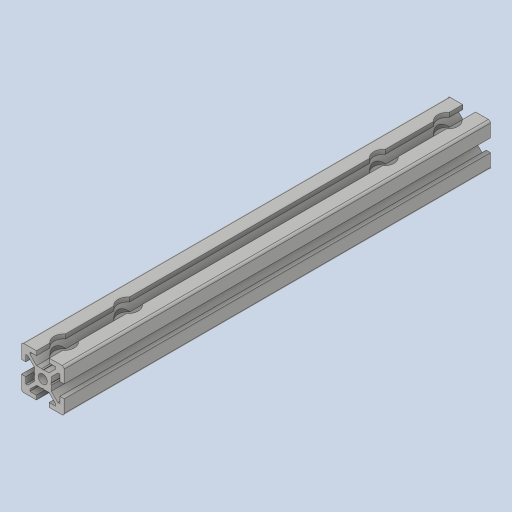
# Autodesk Inventor part: HFS5-2020-200-Z5-XA10-XB40-XC160-XD190
Saved by Autodesk Inventor 2023 (Build 270158000, 158)
## iProperties
Created: 2024-11-09
Part Number: HFS5-2020-200-Z5-XA10-XB40-XC160-XD190
Material: Generic
Catalog Web Link: www.cadenas.de
Description: NFS5-2020, NFSB5-2020, HFS5-2020, HFSB5-2020, CAF5-2020, HFSY5-2020, NFSF5-2020, HFSF5-2020, HFSFB5-2020, NFST5-2020, HFST5-2020, HFSTB5-2020, HFSH5-2020, HFSC5-2020-HFS5 Series Aluminum Extrusions 20 Square -1 Slot-
Vendor: MISUMI
Document SubType Name: Modeling
Designer: psAdmin
Manufacturer: MISUMI
Mass: 35.7548 g
Surface Area: 350.338 cm^2
Volume: 35.7548 cm^3
Density: 1 g/cm^3
Appearance: PSOLRGB-175-175-175
Category: PARTsolutions
Company: MISUMI
PSOL_IDENT_0: {$CADENAS_DATA/23d-libs/misumi/metric/38_al_extrusions_blackets/5/hfs5_2020.prj},727 {VTYP=3D},{NB=H
PSOL_IDENT_1: FS5-2020-200-Z5-XA10-XB40-XC160-XD190},{LINA=HFS5-2020-200-Z5-XA10-XB40-XC160-XD190},{NN=NFS5-2020,
PSOL_IDENT_2: NFSB5-2020, HFS5-2020, HFSB5-2020, CAF5-2020, HFSY5-2020, NFSF5-2020, HFSF5-2020, HFSFB5-2020, NFST5
PSOL_IDENT_3: -2020, HFST5-2020, HFSTB5-2020, HFSH5-2020, HFSC5-2020},{DATE=08.05.2023 08:39:06},{GEOMDATE=27.07.2
PSOL_IDENT_4: 021 03:20:00},{VERSION=},{LINEID=150},{WBVAR=L,ALT1,ALT2,ALT4,ALT5,CP5,DL5,DR5,ALT6,ALT9,ALT10,ALT11
PSOL_IDENT_5: ,HP6,NHL6,DL6,NHR6,DR6,ALT7,ALT8,NH9,AH,BH,CH,DH,EH,NH10,AV,BV,CV,DV,EV,NH11,AP,BP,CP,DP,EP,ALT12,AL
PSOL_IDENT_6: T13,Z,NH12,XA,XB,XC,XD,XE,NH13,YA,YB,YC,YD,YE,ALT16,HP16,DL16,DR16,ALT17,HQ17,JLP,ALT20},{WBNUMERIC=
PSOL_IDENT_7: L,NH9,AH,BH,CH,DH,EH,NH10,AV,BV,CV,DV,EV,NH11,AP,BP,CP,DP,EP,NH12,XA,XB,XC,XD,XE,NH13,YA,YB,YC,YD,YE
PSOL_IDENT_8: ,HQ17,JLP}  {NB=HFS5-2020-200-Z5-XA10-XB40-XC160-XD190},{LINA=HFS5-2020-200-Z5-XA10-XB40-XC160-XD190
PSOL_IDENT_9: },{KT=DUMMY},{PN=HFS5-2020-200-Z5-XA10-XB40-XC160-XD190},{TPS=HFS5-2020},{MAT=A6N01SS-T5 Aluminum Al
PSOL_IDENT_10: loy or 6005A-T5 Aluminum Alloy},{ST=Clear Anodize},{FRMW=20},{FRMH=20},{FRD=4.2},{L=200},{MASS=0.5},
PSOL_IDENT_11: {SA=183},{LX=0.742x10^4},{LY=0.742x10^4},{ALT1=},{M1=0},{DPL1=0},{DPR1=0},{ALT1PN=},{ALT2=},{ALT2ALG=
PSOL_IDENT_12: '','w/o End Tapping (Heli-Coil Insert)','LHP','with LHP (Tapping on the Left (Heli-Coil Insert))','
PSOL_IDENT_13: RHP','with RHP (Tapping on the Right (Heli-Coil Insert))','HPW','with HPW (Tapping on Both Ends (Hel
PSOL_IDENT_14: i-Coil Insert))' },{M2=0},{DP2=0},{ALT2PN=},{ALT4=},{ALT4ALG= '', 'w/o SC (High Precision Cut)', 'SC'
PSOL_IDENT_15: , 'with SC (High Precision Cut)' },{ALT4PN=},{ALT5=},{ALT5ALG= '','w/o 45 Degree Cut','1','with 45 D
PSOL_IDENT_16: egree Cut' },{CP5=},{CP5ALG= '','N/A' },{DL5=},{DL5ALG= '','N/A' },{DR5=},{DR5ALG= '','N/A' },{FRMLA
PSOL_IDENT_17: LT5=0},{FRMRALT5=0},{ALT5PN=},{ALT6=},{ALT6ALG= '','w/o Fastening Location Wrench Access Hole Altera
PSOL_IDENT_18: tions','1','with Fastening Location Wrench Access Hole Alterations' },{ALT9=},{ALT9ALG= '','w/o Loca
PSOL_IDENT_19: tion Specified Wrench Access Hole Alteratons (Horizontal)','1','with Location Specified Wrench Acces
PSOL_IDENT_20: s Hole Alteratons (Horizontal)' },{ALT10=},{ALT10ALG= '','w/o Location Specified Wrench Access Hole
PSOL_IDENT_21: Alteratons (Vertical)','1','with Location Specified Wrench Access Hole Alteratons (Vertical)' },{ALT
PSOL_IDENT_22: 11=},{ALT11ALG= '','w/o Location Specified Wrench Access Hole Alteratons (Crisscross)','1','with Loc
PSOL_IDENT_23: ation Specified Wrench Access Hole Alteratons (Crisscross)' },{HP6=},{HP6ALG= '','N/A' },{NHL6=},{NH
PSOL_IDENT_24: L6ALG= '','N/A' },{DL6=},{DL6ALG= '','N/A' },{NHR6=},{NHR6ALG= '','N/A' },{DR6=},{DR6ALG= '','N/A' }
PSOL_IDENT_25: ,{HL6=0.000},{HL6D=0},{HR6=0.000},{HR6D=0},{J6=0},{J6D=0},{K6=0},{K6D=0},{DD6=0.00},{DD6ALG=0},{ALT7=
PSOL_IDENT_26: },{ALT7ALG= '','N/A' },{ALT8=},{ALT8ALG= '','N/A' },{ALT678PN=},{NH9=0},{NH9MAX=5},{NH9ALG=[0]},{AH=
PSOL_IDENT_27: 0.0},{AHMIN=7},{AHMAX=195},{AHALG=[0]},{BH=0.0},{BHMIN=2},{BHMAX=197},{BHALG=[0]},{CH=0.0},{CHMIN=2}
PSOL_IDENT_28: ,{CHMAX=199},{CHALG=[0]},{DH=0.0},{DHMIN=2},{DHMAX=201},{DHALG=[0]},{EH=0.0},{EHMIN=2},{EHMAX=193},{
PSOL_IDENT_29: EHALG=[0]},{NH10=0},{NH10MAX=5},{NH10ALG=[0]},{AV=0.0},{AVMIN=7},{AVMAX=195},{AVALG=[0]},{BV=0.0},{B
PSOL_IDENT_30: VMIN=2},{BVMAX=197},{BVALG=[0]},{CV=0.0},{CVMIN=2},{CVMAX=199},{CVALG=[0]},{DV=0.0},{DVMIN=2},{DVMAX=
PSOL_IDENT_31: 201},{DVALG=[0]},{EV=0.0},{EVMIN=2},{EVMAX=193},{EVALG=[0]},{NH11=0},{NH11MAX=5},{NH11ALG=[0]},{AP=0
PSOL_IDENT_32: .0},{APMIN=7},{APMAX=195},{APALG=[0]},{BP=0.0},{BPMIN=2},{BPMAX=197},{BPALG=[0]},{CP=0.0},{CPMIN=2},
PSOL_IDENT_33: {CPMAX=199},{CPALG=[0]},{DP=0.0},{DPMIN=2},{DPMAX=201},{DPALG=[0]},{EP=0.0},{EPMIN=2},{EPMAX=193},{E
PSOL_IDENT_34: PALG=[0]},{ALT9PN=},{ALT10PN=},{ALT11PN=},{ALT91011PN=},{ALT12=1},{ALT12ALG= '','w/o Counterbore Hol
PSOL_IDENT_35: e in Specified Position (Vertical)','1','with Counterbore Hole in Specified Position (Vertical)' },{
PSOL_IDENT_36: ALT13=},{ALT13ALG= '','w/o Counterbore Hole in Specified Position (Horizontal)','1','with Counterbor
PSOL_IDENT_37: e Hole in Specified Position (Horizontal)' },{Z=5},{ZALG='5','5','6','6'},{DD12=5.5},{DD112=9.5},{NH
PSOL_IDENT_38: 12=4},{NH12MAX=5},{NH12ALG=[1:5/1]},{XA=10.0},{XAMIN=7},{XAMAX=158.5},{XAALG=[7:158.5/0.5]},{XB=40.0
PSOL_IDENT_39: },{XBMIN=21.5},{XBMAX=170},{XBALG=[21.5:170/0.5]},{XC=160.0},{XCMIN=51.5},{XCMAX=181.5},{XCALG=[51.5
PSOL_IDENT_40: :181.5/0.5]},{XD=190.0},{XDMIN=171.5},{XDMAX=193},{XDALG=[171.5:193/0.5]},{XE=0.0},{XEMIN=201.5},{XE
PSOL_IDENT_41: MAX=193},{XEALG=[0]},{NH13=0},{NH13MAX=5},{NH13ALG=[0]},{YA=0.0},{YAMIN=7},{YAMAX=204.5},{YAALG=[0]}
PSOL_IDENT_42: ,{YB=0.0},{YBMIN=11.5},{YBMAX=216},{YBALG=[0]},{YC=0.0},{YCMIN=11.5},{YCMAX=227.5},{YCALG=[0]},{YD=0
PSOL_IDENT_43: .0},{YDMIN=11.5},{YDMAX=239},{YDALG=[0]},{YE=0.0},{YEMIN=11.5},{YEMAX=193},{YEALG=[0]},{ALT12PN=-XA1
PSOL_IDENT_44: 0-XB40-XC160-XD190},{ALT13PN=},{ALT1213PN=-Z5-XA10-XB40-XC160-XD190},{ALT16=},{ALT16ALG= '','w/o M T
PSOL_IDENT_45: ype Hole Alteration','1','with M Type Hole Alteration' },{HP16=},{HP16ALG= '','N/A' },{DL16=},{DL16A
PSOL_IDENT_46: LG= '','N/A' },{DR16=},{DR16ALG= '','N/A' },{H116=0},{D16=0.0},{ALT16PN=},{ALT17=},{ALT17ALG= '','w/
PSOL_IDENT_47: o L Type Hole Alteration (Top)','1','with L Type Hole Alteration (Top)' },{HQ17=0},{HQ17ALG=0},{JLP=
PSOL_IDENT_48: 0},{JLPMIN=4.9},{JLPMAX=0},{JLPALG=[0]},{L17=0},{D17=0.0},{ALT17PN=},{ALT20=},{ALT20PN=},{ERRORALT01=
PSOL_IDENT_49: OK},{ERRORALT02=OK},{ERRORALT05=OK},{ERRORALT06091=OK},{ERRORALT06092=OK},{ERRORALT06093=OK},{ERRORA
PSOL_IDENT_50: LT06094=OK},{ERRORALT06101=OK},{ERRORALT06102=OK},{ERRORALT06103=OK},{ERRORALT06104=OK},{ERRORALT061
PSOL_IDENT_51: 11=OK},{ERRORALT06112=OK},{ERRORALT06113=OK},{ERRORALT06114=OK},{ERRORALT06121=OK},{ERRORALT06122=OK
PSOL_IDENT_52: },{ERRORALT06123=OK},{ERRORALT06124=OK},{ERRORALT06131=OK},{ERRORALT06132=OK},{ERRORALT06133=OK},{ER
PSOL_IDENT_53: RORALT06134=OK},{ERRORALT0616=OK},{ERRORALT06171=OK},{ERRORALT06172=OK},{ERRORALT06173=OK},{ERRORALT
PSOL_IDENT_54: 0911=OK},{ERRORALT0913=OK},{ERRORALT0916=OK},{ERRORALT0917=OK},{ERRORALT1011=OK},{ERRORALT1012=OK},{
PSOL_IDENT_55: ERRORALT1016=OK},{ERRORALT1017=OK},{ERRORALT1112=OK},{ERRORALT1113=OK},{ERRORALT1116=OK},{ERRORALT11
PSOL_IDENT_56: 17=OK},{ERRORALT1216=OK},{ERRORALT1217=OK},{ERRORALT1316=OK},{ERRORALT1317=OK},{ERRORALT1617=OK},{ER
PSOL_IDENT_57: RORPN=},{TFW=0}
NB: HFS5-2020-200-Z5-XA10-XB40-XC160-XD190
NN: NFS5-2020, NFSB5-2020, HFS5-2020, HFSB5-2020, CAF5-2020, HFSY5-2020, NFSF5-2020, HFSF5-2020, HFSFB5-2020, NFST5-2020, HFST5-2020, HFSTB5-2020, HFSH5-2020, HFSC5-2020
NT: HFS5 Series Aluminum Extrusions 20 Square -1 Slot-
NBSYN: $PN.
LINA: HFS5-2020-200-Z5-XA10-XB40-XC160-XD190
CATALOG: Misumi
PN: HFS5-2020-200-Z5-XA10-XB40-XC160-XD190
TPS: HFS5-2020
MAT: A6N01SS-T5 Aluminum Alloy or 6005A-T5 Aluminum Alloy
ST: Clear Anodize
L: 200
MASS: 0.5
SA: 183
LX: 0.742x10^4
LY: 0.742x10^4
ALT1: w/o End Tapping
M1: 0
DPL1: 0
DPR1: 0
ALT2: w/o End Tapping (Heli-Coil Insert)
M2: 0
DP2: 0
ALT4: w/o SC (High Precision Cut)
ALT5: w/o 45 Degree Cut
CP5: N/A
DL5: N/A
DR5: N/A
ALT6: w/o Fastening Location Wrench Access Hole Alterations
ALT9: w/o Location Specified Wrench Access Hole Alteratons (Horizontal)
ALT10: w/o Location Specified Wrench Access Hole Alteratons (Vertical)
ALT11: w/o Location Specified Wrench Access Hole Alteratons (Crisscross)
HP6: N/A
NHL6: N/A
DL6: N/A
NHR6: N/A
DR6: N/A
HL6D: 0
HR6D: 0
J6D: 0
K6D: 0
DD6: 0
ALT7: N/A
ALT8: N/A
NH9: 0
AH: 0
BH: 0
CH: 0
DH: 0
EH: 0
NH10: 0
AV: 0
BV: 0
CV: 0
DV: 0
EV: 0
NH11: 0
AP: 0
BP: 0
CP: 0
DP: 0
EP: 0
ALT12: with Counterbore Hole in Specified Position (Vertical)
ALT13: w/o Counterbore Hole in Specified Position (Horizontal)
Z: 5
DD12: 5.5
DD112: 9.5
NH12: 4
XA: 10
XB: 40
XC: 160
XD: 190
XE: 0
NH13: 0
YA: 0
YB: 0
YC: 0
YD: 0
YE: 0
ALT16: w/o M Type Hole Alteration
HP16: N/A
DL16: N/A
DR16: N/A
H116: 0
D16: 0
ALT17: w/o L Type Hole Alteration (Top)
HQ17: 0
JLP: 0
D17: 0
ALT20: w/o CW (End Face C Chamfering)
SUPPLIER: MISUMI
ARTICLENO: HFS5-2020-200-Z5-XA10-XB40-XC160-XD190
BOMINFO: HFS5-2020-200-Z5-XA10-XB40-XC160-XD190
CREATOR: CADENAS GmbH
Title: HFS5-2020-200-Z5-XA10-XB40-XC160-XD190
Author: Cadenas PARTsolutions
Comments: HFS5 Series Aluminum Extrusions 20 Square -1 Slot-
Autodesk Inventor part; units mm, degrees
sketch "Sketch_1" plane through (0, 0, 0) normal (0, 0, 1) x (1, 0, 0)
  line L0 (-10, -3) -> (-10, -9)
  arc A0 (-10, -9) -> (-9, -10) centre (-9, -9) ccw
  line L1 (-9, -10) -> (-3, -10)
  line L2 (-3, -10) -> (-3, -8)
  line L3 (-3, -8) -> (-6, -8)
  line L4 (-6, -8) -> (-6, -7.0607)
  line L5 (-6, -7.0607) -> (-2.9393, -4)
  line L6 (-2.9393, -4) -> (-0.5196, -4)
  line L7 (-0.5196, -4) -> (0, -3.7)
  line L8 (0, -3.7) -> (0.5196, -4)
  line L9 (0.5196, -4) -> (2.9393, -4)
  line L10 (2.9393, -4) -> (6, -7.0607)
  line L11 (6, -7.0607) -> (6, -8)
  line L12 (6, -8) -> (3, -8)
  line L13 (3, -8) -> (3, -10)
  line L14 (3, -10) -> (9, -10)
  arc A1 (9, -10) -> (10, -9) centre (9, -9) ccw
  line L15 (10, -9) -> (10, -3)
  line L16 (10, -3) -> (8, -3)
  line L17 (8, -3) -> (8, -6)
  line L18 (8, -6) -> (7.0607, -6)
  line L19 (7.0607, -6) -> (4, -2.9393)
  line L20 (4, -2.9393) -> (4, -0.5196)
  line L21 (4, -0.5196) -> (3.7, 0)
  line L22 (3.7, 0) -> (4, 0.5196)
  line L23 (4, 0.5196) -> (4, 2.9393)
  line L24 (4, 2.9393) -> (7.0607, 6)
  line L25 (7.0607, 6) -> (8, 6)
  line L26 (8, 6) -> (8, 3)
  line L27 (8, 3) -> (10, 3)
  line L28 (10, 3) -> (10, 9)
  arc A2 (10, 9) -> (9, 10) centre (9, 9) ccw
  line L29 (9, 10) -> (3, 10)
  line L30 (3, 10) -> (3, 8)
  line L31 (3, 8) -> (6, 8)
  line L32 (6, 8) -> (6, 7.0607)
  line L33 (6, 7.0607) -> (2.9393, 4)
  line L34 (2.9393, 4) -> (0.5196, 4)
  line L35 (0.5196, 4) -> (0, 3.7)
  line L36 (0, 3.7) -> (-0.5196, 4)
  line L37 (-0.5196, 4) -> (-2.9393, 4)
  line L38 (-2.9393, 4) -> (-6, 7.0607)
  line L39 (-6, 7.0607) -> (-6, 8)
  line L40 (-6, 8) -> (-3, 8)
  line L41 (-3, 8) -> (-3, 10)
  line L42 (-3, 10) -> (-9, 10)
  arc A3 (-9, 10) -> (-10, 9) centre (-9, 9) ccw
  line L43 (-10, 9) -> (-10, 3)
  line L44 (-10, 3) -> (-8, 3)
  line L45 (-8, 3) -> (-8, 6)
  line L46 (-8, 6) -> (-7.0607, 6)
  line L47 (-7.0607, 6) -> (-4, 2.9393)
  line L48 (-4, 2.9393) -> (-4, 0.5196)
  line L49 (-4, 0.5196) -> (-3.7, 0)
  line L50 (-3.7, 0) -> (-4, -0.5196)
  line L51 (-4, -0.5196) -> (-4, -2.9393)
  line L52 (-4, -2.9393) -> (-7.0607, -6)
  line L53 (-7.0607, -6) -> (-8, -6)
  line L54 (-8, -6) -> (-8, -3)
  line L55 (-8, -3) -> (-10, -3)
  constraints: 112 end point, 8 point on circle, 4 centre point
extrude "Extrusion1" add sketch "Sketch_1" against normal blind 200
sketch "Sketch2" plane through (0, 0, -200) normal (0, 0, -1) x (-1, 0, 0)
  point P0 (0, 0)
hole "Hole1" at (0, 0, -200) direction (0, 0, 1) diameter 4.2 depth 200
sketch "Sketch_30" plane through (0, 0, 0) normal (1, 0, 0) x (0, 0, -1)
  line L0 (10, -10) -> (10, 10)
  line L1 (10, 10) -> (14.75, 10)
  line L2 (14.75, 10) -> (14.75, 4)
  line L3 (14.75, 4) -> (12.75, 4)
  line L4 (12.75, 4) -> (12.75, -10)
  line L5 (12.75, -10) -> (10, -10)
  line L6 (10, -10) -> (10, 10)
  constraints: 14 end point
revolve "Revolution1" cut sketch "Sketch_30" angle 360 about axis through (0, -10, -10) along (0, -1, 0)
sketch "Sketch_31" plane through (0, 0, 0) normal (1, 0, 0) x (0, 0, -1)
  line L0 (40, -10) -> (40, 10)
  line L1 (40, 10) -> (44.75, 10)
  line L2 (44.75, 10) -> (44.75, 4)
  line L3 (44.75, 4) -> (42.75, 4)
  line L4 (42.75, 4) -> (42.75, -10)
  line L5 (42.75, -10) -> (40, -10)
  line L6 (40, -10) -> (40, 10)
  constraints: 14 end point
revolve "Revolution2" cut sketch "Sketch_31" angle 360 about axis through (0, -10, -40) along (0, -1, 0)
sketch "Sketch_47" plane through (0, 0, 0) normal (1, 0, 0) x (0, 0, -1)
  line L0 (160, -10) -> (160, 10)
  line L1 (160, 10) -> (164.75, 10)
  line L2 (164.75, 10) -> (164.75, 4)
  line L3 (164.75, 4) -> (162.75, 4)
  line L4 (162.75, 4) -> (162.75, -10)
  line L5 (162.75, -10) -> (160, -10)
  line L6 (160, -10) -> (160, 10)
  constraints: 14 end point
revolve "Revolution3" cut sketch "Sketch_47" angle 360 about axis through (0, -10, -160) along (0, -1, 0)
sketch "Sketch_48" plane through (0, 0, 0) normal (1, 0, 0) x (0, 0, -1)
  line L0 (190, -10) -> (190, 10)
  line L1 (190, 10) -> (194.75, 10)
  line L2 (194.75, 10) -> (194.75, 4)
  line L3 (194.75, 4) -> (192.75, 4)
  line L4 (192.75, 4) -> (192.75, -10)
  line L5 (192.75, -10) -> (190, -10)
  line L6 (190, -10) -> (190, 10)
  constraints: 14 end point
revolve "Revolution4" cut sketch "Sketch_48" angle 360 about axis through (0, -10, -190) along (0, -1, 0)
ref_plane "C1_XY" through (0, 0, 0) normal (0, 0, 1) x (1, 0, 0)
ref_plane "C1_YZ" through (0, 0, 0) normal (1, 0, 0) x (0, 1, 0)
ref_plane "C1_ZX" through (0, 0, 0) normal (0, 1, 0) x (0, 0, 1)
body "Solid1"
